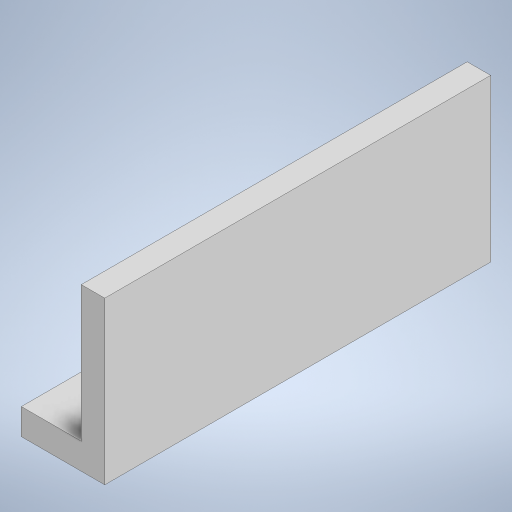
# Autodesk Inventor part: pecinha_empunhadura
Saved by Autodesk Inventor 2024.3 (Build 283343000, 343)
## iProperties
Created: 2024-12-01
Part Number: pecinha_empunhadura
Material: Genérico
Document SubType Name: Modeling
Designer: lostv
Density: 1 g/cm^3
Appearance: Padrão
Author: lostv
Autodesk Inventor part; units mm, degrees
ref_plane "YZ Plane" through (0, 0, 0) normal (1, 0, 0) x (0, 1, 0)
ref_plane "XZ Plane" through (0, 0, 0) normal (0, 1, 0) x (-1, 0, 0)
ref_plane "XY Plane" through (0, 0, 0) normal (0, 0, 1) x (1, 0, 0)
sketch "Esboço1" plane through (0, 0, 0) normal (0, 1, 0) x (-1, 0, 0)
  line L0 (11.8731, -18.4543) -> (11.8731, 18.5457)
  line L1 (11.8731, 18.5457) -> (19.8731, 18.5457)
  line L2 (19.8731, 18.5457) -> (19.8731, -18.4543)
  line L3 (19.8731, -18.4543) -> (11.8731, -18.4543)
  line L4 (11.8731, -18.4543) -> (11.8731, 18.5457)
  circle A0 centre (15.8731, 12.5457) radius 1.5
  circle A1 centre (15.8731, -12.4543) radius 1.5
  line L5 (14.1231, -18.4543) -> (14.1231, 18.5457)
  point P0 (15.8731, 18.5457)
  point P1 (15.8731, -18.4543)
  dimension "d2" = 8
  dimension "d3" = 3
  dimension "d5" = 6
  dimension "d6" = 6
  dimension "d8" = 4
  dimension "d9" = 2.25
  dimension "d10" = 3
  constraints: 12 end point, 2 centre point, 2 midpoint, 2 parallel, 2 point on line, 1 horizontal, 1 perpendicular, 1 vertical
  measures "d2" distance of L3.start L3.end
  measures "d3" diameter of A0
  measures "d5" distance of point (15.873, 18.546) A0.centre
  measures "d6" distance of point (15.873, -18.454) A1.centre
  measures "d8" distance from line of L2 A0.centre
  measures "d9" distance between parallel lines of L0 L5
  measures "d10" diameter of A1
extrude "Extrusão1" add sketch "Esboço1" along normal blind 2.5 contours L5 L1 L2 L3
extrude "Extrusão2" add sketch "Esboço1" along normal blind 15.5 contours L0 L1 L5 L3
